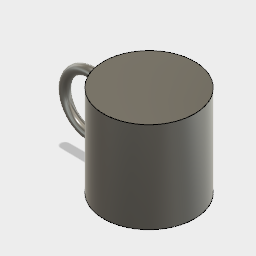
FPROJ_4 (Autodesk Fusion 360 design; units mm, degrees)
Autodesk Fusion 360 part; units mm, degrees
cylinder "圆柱体基本要素1" add diameter 20 height 20 placed x (1, 0, 0) y (0, 0, -1) z (0, 1, 0) at (0, 0, 0) makes body 1
cylinder "圆柱体基本要素2" add diameter 18 height 20 placed x (1, 0, 0) y (0, 0, -1) z (0, 1, 0) at (25, 0, -20) separate body makes body 2
torus "圆环体基本要素2" add centre line diameter 12 section diameter 2 placed x (1, 0, 0) y (0, 0, -1) z (0, 1, 0) at (-25, 0, 50) separate body makes body 3
move_body "MoveFace1" bodies 3 to x (-0.985554, 0.154148, 0.070157) y (0.066656, -0.027772, 0.997389) z (0.155694, 0.987657, 0.017095) at (-43.7543, -34.6312, -0.942) on bodies 3
move_body "MoveFace2" bodies 3 to x (0.996758, 0.001351, 0.080452) y (0.001351, 0.999437, -0.033519) z (-0.080452, 0.033519, 0.996195) at (-1.1237, 0.0832, 3.4482) on bodies 3
combine "合并1" operation add target body 3 tool bodies 1
move_body "对齐1" bodies 3 to x (1, 0, 0) y (0, 1, 0) z (0, 0, 1) at (0, 0, 0)
move_body "移动1" bodies 2 to x (1, 0, 0) y (0, 1, 0) z (0, 0, 1) at (-29.4924, 24.2451, 0)
move_body "移动2" bodies 2 to x (1, 0, 0) y (0, 1, 0) z (0, 0, 1) at (6.0304, 0, 23.8223)
move_face "MoveFace3" to x (1, 0, 0) y (0, 1, 0) z (0, 0, 1) at (-4.4713, -1.4024, -1.0547) 1 faces at (10.4933, 37.5784, 4.7184) on bodies 2
move_body "移动3" bodies 2 to x (1, 0, 0) y (0, 1, 0) z (0, 0, 1) at (0, -0.618, -1.8927)
move_body "移动4" bodies 2 to x (1, 0, 0) y (0, 1, 0) z (0, 0, 1) at (3, 0, 0)
move_body "移动5" bodies 2 to x (1, 0, 0) y (0, 1, 0) z (0, 0, 1) at (0, 0, -1)
move_body "对齐2" bodies 3 to x (1, 0, 0) y (0, 1, 0) z (0, 0, 1) at (0, 23.6271, 0)
move_face "偏移面1" offset -2 1 faces at (2.097, 43.6271, -1.8151) on bodies 2
combine "合并2" operation cut target body 3 tool bodies 2
